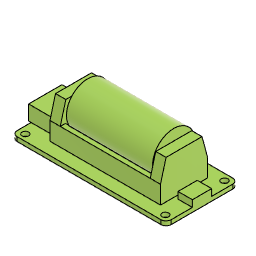
NRF_RC_Case_ESP32 v14 (Autodesk Fusion 360 archive; units mm, degrees)
design "SMARS-myMOD_16340 Sheild"
Autodesk Fusion 360 part; units mm, degrees
sketch "Sketch1" plane through (0, 0, 0) normal (0, 0, 1) x (1, 0, 0)
  line L0 (2, 0) -> (58, 0)
  line L1 (60, 2) -> (60, 26)
  line L2 (58, 28) -> (2, 28)
  line L3 (0, 26) -> (0, 2)
  arc A0 (2, 28) -> (0, 26) centre (2, 26) ccw
  arc A1 (60, 26) -> (58, 28) centre (58, 26) ccw
  arc A2 (58, 0) -> (60, 2) centre (58, 2) ccw
  arc A3 (0, 2) -> (2, 0) centre (2, 2) ccw
  point P0 (60, 0)
  point P1 (0, 28)
  dimension "d56" = 60
  dimension "d57" = 28
  dimension "d58" = 2
  constraint horizontal L0
  constraint vertical L1
  constraint horizontal L2
  constraint vertical L3
  constraint coincident P1 L2
  constraint coincident P1 L3
  constraint tangent L2 A0
  constraint tangent L3 A0
  constraint tangent L1 A1
  constraint tangent L2 A1
  constraint equal A0 A1
  constraint coincident P0 L0
  constraint coincident P0 L1
  constraint tangent L0 A2
  constraint tangent L1 A2
  constraint equal A0 A2
  constraint coincident origin L0
  constraint coincident origin L3
  constraint tangent L0 A3
  constraint tangent L3 A3
  constraint equal A0 A3
  measures "d56" distance of origin P0
  measures "d57" distance of origin P1
  measures "d58" radius of A0
extrude "Extrude1" add sketch "Sketch1" along normal blind 1.65
sketch "Sketch2" plane through (0, 0, 1.65) normal (0, 0, 1) x (-1, 0, 0)
  arc A0 (0, -2) -> (-2, 0) centre (-2, -2) ccw
  line L0 (-2, 0) -> (-58, 0)
  arc A1 (-58, 0) -> (-60, -2) centre (-58, -2) ccw
  line L1 (-60, -2) -> (-60, -26)
  arc A2 (-60, -26) -> (-58, -28) centre (-58, -26) ccw
  line L2 (-58, -28) -> (-2, -28)
  arc A3 (-2, -28) -> (0, -26) centre (-2, -26) ccw
  line L3 (0, -26) -> (0, -2)
  line L4 (1, -20.5) -> (-9, -20.5)
  line L5 (-9, -20.5) -> (-9, -7.5)
  line L6 (-9, -7.5) -> (1, -7.5)
  line L7 (1, -7.5) -> (1, -20.5)
  line L8 (0, -14) -> (-60, -14) construction
  dimension "d61" = 10
  dimension "d62" = 13
  dimension "d63" = 1
  constraint horizontal L4
  constraint vertical L5
  constraint horizontal L6
  constraint vertical L7
  constraint midpoint L3 L8.start
  constraint midpoint L1 L8.end
  constraint symmetric L4 L6 L8
  measures "d61" distance of L4.start L4.end
  measures "d62" distance of L4.start L6.end
  measures "d63" distance of L3 L7
extrude "Extrude2" add sketch "Sketch2" along normal blind 5.75 contours L3 L4 L6 L7 | L3 L4 L5 L6
sketch "Sketch3" plane through (0, 0, 1.65) normal (0, 0, 1) x (-1, 0, 0)
  line L0 (-9, -7.5) -> (0, -7.5)
  line L1 (0, -7.5) -> (0, -2)
  arc A0 (0, -2) -> (-2, 0) centre (-2, -2) ccw
  line L2 (-2, 0) -> (-58, 0)
  arc A1 (-58, 0) -> (-60, -2) centre (-58, -2) ccw
  line L3 (-60, -2) -> (-60, -26)
  arc A2 (-60, -26) -> (-58, -28) centre (-58, -26) ccw
  line L4 (-58, -28) -> (-2, -28)
  arc A3 (-2, -28) -> (0, -26) centre (-2, -26) ccw
  line L5 (0, -26) -> (0, -20.5)
  line L6 (0, -20.5) -> (-9, -20.5)
  line L7 (-9, -20.5) -> (-9, -7.5)
  line L8 (-9, -14) -> (-60, -14) construction
  line L9 (-10, -23.15) -> (-53, -23.15)
  line L10 (-53, -23.15) -> (-53, -4.85)
  line L11 (-53, -4.85) -> (-10, -4.85)
  line L12 (-10, -4.85) -> (-10, -23.15)
  dimension "d66" = 43
  dimension "d67" = 18.3
  dimension "d68" = 1
  constraint midpoint L7 L8.start
  constraint midpoint L3 L8.end
  constraint horizontal L9
  constraint vertical L10
  constraint horizontal L11
  constraint vertical L12
  constraint symmetric L8 L9 L11
  measures "d66" distance of L9.start L9.end
  measures "d67" distance of L9.start L11.end
  measures "d68" distance of L7 L12
extrude "Extrude3" add sketch "Sketch3" along normal blind 15 contours L9 L10 L11 L12
sketch "Sketch4" plane through (53, 0, 0) normal (1, 0, 0) x (0, 1, 0)
  line L0 (4.85, 1.65) -> (23.15, 1.65)
  line L1 (23.15, 1.65) -> (23.15, 16.65)
  line L2 (23.15, 16.65) -> (4.85, 16.65)
  line L3 (4.85, 16.65) -> (4.85, 1.65)
  line L4 (4.85, 8.65) -> (7.2688, 17.65)
  line L5 (7.2688, 17.65) -> (20.7313, 17.65)
  line L6 (20.7313, 17.65) -> (23.15, 8.65)
  line L7 (4.85, 8.65) -> (23.15, 8.65) construction
  line L8 (7, 16.65) -> (21, 16.65) construction
  line L9 (14, 16.65) -> (14, 1.65) construction
  dimension "d71" = 14
  dimension "d72" = 7
  dimension "d73" = 1
  constraint coincident L3 L4.start
  constraint perpendicular L3 L5
  constraint coincident L1 L6.end
  constraint horizontal L7
  constraint coincident L4 L8.start
  constraint coincident L2 L8.start
  constraint coincident L6 L8.end
  constraint coincident L2 L8.end
  constraint midpoint L8 L9.start
  constraint midpoint L0 L9.end
  constraint symmetric L8.start L8.end L9
  measures "d71" distance of L8.start L8.end
  measures "d72" distance of L0 L7
  measures "d73" distance of L2 L5
extrude "Extrude4" cut sketch "Sketch4" against normal up to surface (43 mm away) contours L2 L3 L4 | L1 L2 L6
sketch "Sketch5" plane through (0, 4.85, 0) normal (0, -1, 0) x (1, 0, 0)
  line L0 (53, 8.65) -> (10, 8.65)
  line L1 (10, 8.65) -> (10, 1.65)
  line L2 (10, 1.65) -> (53, 1.65)
  line L3 (53, 1.65) -> (53, 8.65)
  line L4 (14, 16.65) -> (49, 16.65)
  line L5 (49, 16.65) -> (49, 8.65)
  line L6 (49, 8.65) -> (14, 8.65)
  line L7 (14, 8.65) -> (14, 16.65)
  line L8 (10, 8.65) -> (10, 16.65)
  line L9 (31.5, 1.65) -> (31.5, 16.653) construction
  line L10 (10, 16.65) -> (53, 16.65) construction
  dimension "d76" = 4
  constraint horizontal L4
  constraint vertical L5
  constraint horizontal L6
  constraint vertical L7
  constraint midpoint L2 L9.start
  constraint perpendicular L4 L9
  constraint symmetric L5 L7 L9
  constraint collinear L0 L6
  constraint collinear L4 L10
  measures "d76" distance of L7 L8
extrude "Extrude5" cut sketch "Sketch5" against normal through all contours L0 L4 L5 L6 L7
sketch "Sketch6" plane through (0, 0, 8.65) normal (0, 0, 1) x (-1, 0, 0)
  line L0 (-49, -23.15) -> (-14, -23.15)
  line L1 (-14, -23.15) -> (-14, -4.85)
  line L2 (-14, -4.85) -> (-49, -4.85)
  line L3 (-49, -4.85) -> (-49, -23.15)
  line L4 (-14, -14) -> (-49, -14) construction
  line L5 (-14, -21.15) -> (-49, -21.15)
  line L6 (-49, -21.15) -> (-49, -6.85)
  line L7 (-49, -6.85) -> (-14, -6.85)
  line L8 (-14, -6.85) -> (-14, -21.15)
  dimension "d78" = 2
  constraint midpoint L1 L4.start
  constraint midpoint L3 L4.end
  constraint horizontal L5
  constraint vertical L6
  constraint horizontal L7
  constraint vertical L8
  constraint coincident L3 L6.end
  constraint coincident L1 L5.start
  constraint symmetric L4 L5 L7
  measures "d78" distance of L0 L5
extrude "Extrude6" cut sketch "Sketch6" against normal blind 6 contours L1 L3 L5 L6 L7 L8
sketch "Sketch7" plane through (49, 0, 0) normal (-1, 0, 0) x (0, -1, 0)
  line L0 (-4.85, 8.65) -> (-7, 16.65)
  line L1 (-7, 16.65) -> (-21, 16.65)
  line L2 (-21, 16.65) -> (-23.15, 8.65)
  line L3 (-23.15, 8.65) -> (-21.15, 8.65)
  line L4 (-21.15, 8.65) -> (-21.15, 2.65)
  line L5 (-21.15, 2.65) -> (-6.85, 2.65)
  line L6 (-6.85, 2.65) -> (-6.85, 8.65)
  line L7 (-6.85, 8.65) -> (-4.85, 8.65)
  line L8 (-14, 16.65) -> (-14, 2.65) construction
  circle A0 centre (-14, 12.65) radius 8.25
  dimension "d81" = 16.5
  dimension "d82" = 4
  constraint midpoint L1 L8.start
  constraint midpoint L5 L8.end
  constraint coincident L8 A0.centre
  measures "d81" diameter of A0
  measures "d82" distance of L1 A0.centre
extrude "Extrude7" add sketch "Sketch7" along normal blind 33.5 contours L0 L1 L2 L3 L4 L6 L7 A0 | L0 L1 L2 A0
sketch "Sketch8" plane through (0, 0, 1.65) normal (0, 0, 1) x (-1, 0, 0)
  line L0 (-10, -4.85) -> (-10, -23.15)
  line L1 (-10, -23.15) -> (-53, -23.15)
  line L2 (-53, -23.15) -> (-53, -4.85)
  line L3 (-53, -4.85) -> (-10, -4.85)
  line L4 (-9, -7.5) -> (0, -7.5)
  line L5 (0, -7.5) -> (0, -2)
  arc A0 (0, -2) -> (-2, 0) centre (-2, -2) ccw
  line L6 (-2, 0) -> (-58, 0)
  arc A1 (-58, 0) -> (-60, -2) centre (-58, -2) ccw
  line L7 (-60, -2) -> (-60, -26)
  arc A2 (-60, -26) -> (-58, -28) centre (-58, -26) ccw
  line L8 (-58, -28) -> (-2, -28)
  arc A3 (-2, -28) -> (0, -26) centre (-2, -26) ccw
  line L9 (0, -26) -> (0, -20.5)
  line L10 (0, -20.5) -> (-9, -20.5)
  line L11 (-9, -20.5) -> (-9, -7.5)
  line L12 (-60, -14) -> (-9, -14) construction
  line L13 (-60, -17.75) -> (-54.4, -17.75)
  line L14 (-54.4, -17.75) -> (-54.4, -10.25)
  line L15 (-54.4, -10.25) -> (-60, -10.25)
  line L16 (-60, -10.25) -> (-60, -17.75)
  dimension "d85" = 5.6
  dimension "d86" = 7.5
  constraint midpoint L7 L12.start
  constraint midpoint L11 L12.end
  constraint horizontal L13
  constraint vertical L14
  constraint horizontal L15
  constraint vertical L16
  constraint coincident L7 L13.start
  constraint symmetric L12 L13 L15
  measures "d85" distance of L13.start L13.end
  measures "d86" distance of L13.start L15.end
extrude "Extrude8" add sketch "Sketch8" along normal blind 2.6 contours L7 L13 L14 L15 L16
sketch "Sketch9" plane through (0, 0, 0) normal (0, 0, -1) x (1, 0, 0)
  arc A0 (2, 0) -> (0, -2) centre (2, -2) ccw
  line L0 (0, -2) -> (0, -26)
  arc A1 (0, -26) -> (2, -28) centre (2, -26) ccw
  line L1 (2, -28) -> (58, -28)
  arc A2 (58, -28) -> (60, -26) centre (58, -26) ccw
  line L2 (60, -26) -> (60, -2)
  arc A3 (60, -2) -> (58, 0) centre (58, -2) ccw
  line L3 (58, 0) -> (2, 0)
  line L4 (0, -14) -> (60, -14) construction
  line L5 (30, 0) -> (30, -28) construction
  circle A4 centre (2.75, -2.5) radius 1.3
  circle A5 centre (57.25, -2.5) radius 1.3
  circle A6 centre (2.75, -25.5) radius 1.3
  circle A7 centre (57.25, -25.5) radius 1.3
  line L6 (2.75, -2.5) -> (57.25, -2.5) construction
  line L7 (57.25, -2.5) -> (57.25, -25.5) construction
  line L8 (57.25, -25.5) -> (2.75, -25.5) construction
  line L9 (2.75, -25.5) -> (2.75, -2.5) construction
  dimension "d89" = 23
  dimension "d90" = 54.5
  dimension "d91" = 2.6
  constraint midpoint L0 L4.start
  constraint midpoint L2 L4.end
  constraint midpoint L3 L5.start
  constraint midpoint L1 L5.end
  constraint coincident A4.centre L6.start
  constraint coincident A5.centre L6.end
  constraint horizontal L6
  constraint coincident A7.centre L7.end
  constraint perpendicular L4 L7
  constraint coincident A6.centre L8.end
  constraint perpendicular L7 L8
  constraint perpendicular L6 L9
  constraint symmetric L4 L6 L8
  constraint symmetric L5 L7 L9
  constraint equal A4 A6
  constraint equal A5 A7
  constraint equal A6 A7
  measures "d89" distance of A5.centre A7.centre
  measures "d90" distance of A4.centre A5.centre
  measures "d91" diameter of A4
extrude "Extrude9" cut sketch "Sketch9" against normal up to surface (1.65 mm away) contours A4 | A5 | A6 | A7
sketch "Sketch10" plane through (0, 0, 1.65) normal (0, 0, 1) x (-1, 0, 0)
  circle A0 centre (-57.25, -2.5) radius 1.3
  circle A1 centre (-57.25, -25.5) radius 1.3
  circle A2 centre (-2.75, -2.5) radius 1.3
  circle A3 centre (-2.75, -25.5) radius 1.3
  line L0 (-54.4, -17.75) -> (-60, -17.75)
  line L1 (-60, -17.75) -> (-60, -26)
  arc A4 (-60, -26) -> (-58, -28) centre (-58, -26) ccw
  line L2 (-58, -28) -> (-2, -28)
  arc A5 (-2, -28) -> (0, -26) centre (-2, -26) ccw
  line L3 (0, -26) -> (0, -20.5)
  line L4 (0, -20.5) -> (-9, -20.5)
  line L5 (-9, -20.5) -> (-9, -7.5)
  line L6 (-9, -7.5) -> (0, -7.5)
  line L7 (0, -7.5) -> (0, -2)
  arc A6 (0, -2) -> (-2, 0) centre (-2, -2) ccw
  line L8 (-2, 0) -> (-58, 0)
  arc A7 (-58, 0) -> (-60, -2) centre (-58, -2) ccw
  line L9 (-60, -2) -> (-60, -10.25)
  line L10 (-60, -10.25) -> (-54.4, -10.25)
  line L11 (-54.4, -10.25) -> (-54.4, -17.75)
  line L12 (-10, -4.85) -> (-10, -23.15)
  line L13 (-10, -23.15) -> (-53, -23.15)
  line L14 (-53, -23.15) -> (-53, -4.85)
  line L15 (-53, -4.85) -> (-10, -4.85)
  line L16 (-6.4, -28) -> (-15.3, -28)
  line L17 (-15.3, -28) -> (-15.3, -24.4)
  line L18 (-15.3, -24.4) -> (-6.4, -24.4)
  line L19 (-6.4, -24.4) -> (-6.4, -28)
  dimension "d1" = 8.9
  dimension "d2" = 3.6
  dimension "d3" = 15.3
  constraint horizontal L16
  constraint vertical L17
  constraint horizontal L18
  constraint vertical L19
  constraint coincident L2 L16.start
  measures "d1" distance of L16.start L16.end
  measures "d2" distance of L16.start L18.end
  measures "d3" distance of L3 L17
extrude "Extrude10" add sketch "Sketch10" along normal blind 3.6 contours L2 L16 L17 L18 L19
sketch "Sketch11" plane through (0, 28, 0) normal (0, 1, 0) x (-1, 0, 0)
  line L0 (-58, 0) -> (-2, 0)
  line L1 (-2, 0) -> (-2, 1.65)
  line L2 (-2, 1.65) -> (-6.4, 1.65)
  line L3 (-6.4, 1.65) -> (-6.4, 5.25)
  line L4 (-6.4, 5.25) -> (-15.3, 5.25)
  line L5 (-15.3, 5.25) -> (-15.3, 1.65)
  line L6 (-15.3, 1.65) -> (-58, 1.65)
  line L7 (-58, 1.65) -> (-58, 0)
  line L8 (-15.3, 3.45) -> (-6.4, 3.45) construction
  line L9 (-8.9, 2.7) -> (-10.4, 2.7)
  line L10 (-10.4, 2.7) -> (-10.4, 4.2)
  line L11 (-10.4, 4.2) -> (-8.9, 4.2)
  line L12 (-8.9, 4.2) -> (-8.9, 2.7)
  line L13 (-8.9, 2.7) -> (-10.4, 4.2) construction
  line L14 (-10.4, 2.7) -> (-8.9, 4.2) construction
  point P0 (-9.65, 3.45)
  dimension "d6" = 1.5
  dimension "d7" = 1.5
  dimension "d8" = 2.5
  constraint midpoint L5 L8.start
  constraint midpoint L3 L8.end
  constraint horizontal L9
  constraint perpendicular L9 L10
  constraint parallel L9 L11
  constraint parallel L10 L12
  constraint coincident L13 P0
  constraint coincident L14 P0
  constraint coincident L8 P0
  measures "d6" distance of L10.end L11.end
  measures "d7" distance of L9.end L10.end
  measures "d8" distance of L3 L12
extrude "Extrude11" add sketch "Sketch11" along normal blind 3.4 contours L9 L10 L11 L12
